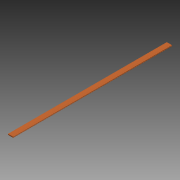
# Autodesk Inventor part: TimberTech
Saved by Autodesk Inventor 2015 (Build 190159000, 159)
## iProperties
Created: 2014-05-27
Part Number: TimberTech
Material: Polyethylene, High Density
Document SubType Name: Modeling
Designer: Haden
Density: 0.952 g/cm^3
Appearance: Cherry - Natural Low Gloss
Mass: 13133.3 g
Surface Area: 14091.5 cm^2
Volume: 13795.5 cm^3
Author: Haden
Autodesk Inventor part; units mm, degrees
ref_plane "YZ Plane" through (0, 0, 0) normal (1, 0, 0) x (0, 1, 0)
ref_plane "XZ Plane" through (0, 0, 0) normal (0, 1, 0) x (-1, 0, 0)
ref_plane "XY Plane" through (0, 0, 0) normal (0, 0, 1) x (1, 0, 0)
sketch "Sketch1" plane through (0, 0, 0) normal (0, 0, 1) x (1, 0, 0)
  line L0 (3.175, 0) -> (132.969, 0)
  line L1 (132.969, -23.876) -> (3.175, -23.876)
  line L2 (0, -9.525) -> (6.35, -9.525)
  line L3 (6.35, -9.525) -> (6.35, -15.875)
  line L4 (6.35, -15.875) -> (0, -15.875)
  line L5 (136.144, -9.525) -> (129.794, -9.525)
  line L6 (129.794, -9.525) -> (129.794, -15.875)
  line L7 (129.794, -15.875) -> (136.144, -15.875)
  line L8 (0, -20.701) -> (0, -15.875)
  line L9 (0, -9.525) -> (0, -3.175)
  line L10 (136.144, -3.175) -> (136.144, -9.525)
  line L11 (136.144, -15.875) -> (136.144, -20.701)
  arc A0 (3.175, 0) -> (0, -3.175) centre (3.175, -3.175) ccw
  arc A1 (0, -20.701) -> (3.175, -23.876) centre (3.175, -20.701) ccw
  arc A2 (136.144, -3.175) -> (132.969, 0) centre (132.969, -3.175) ccw
  arc A3 (132.969, -23.876) -> (136.144, -20.701) centre (132.969, -20.701) ccw
  point P0 (0, 0)
  point P1 (136.144, -23.876)
  point P2 (136.144, 0)
  point P3 (0, -23.876)
  dimension "d0" = 136.144
  dimension "d1" = 23.876
  dimension "d3" = 6.35
  dimension "d4" = 9.525
  dimension "d5" = 3.175
  constraints: 24 end point, 8 perpendicular, 8 point on circle, 8 point on line, 8 tangent, 5 parallel, 4 centre point, 3 collinear, 3 equal length, 3 equal radius, 3 horizontal
  measures "d0" distance of point (136.144, -23.876) point (0, -23.876)
  measures "d1" distance of point (136.144, 0) point (136.144, -23.876)
  measures "d3" distance of L2.end L3.end
  measures "d4" distance between parallel lines of L0 L2
  measures "d5" radius of A0
extrude "Extrusion1" add sketch "Sketch1" along normal blind 4064
body "Solid1"
